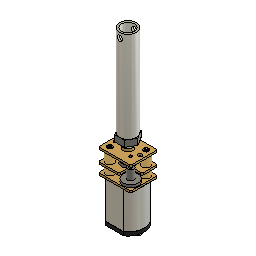
MicroGearMotor v14 (Autodesk Fusion 360 design; units mm, degrees)
Autodesk Fusion 360 part; units mm, degrees
note: some values were not read from the file. Chosen so that the rebuilt part matches the saved one: which bodies a step acts on; which face or edge a step refers to; how an offset face is resized; where a step starts. Set by a fixed rule: which sketch regions a step uses.
sketch "Sketch1" plane through (0, 0, 0) normal (0, 1, 0) x (1, 0, 0) in component "GearboxScaffolding"
  line L0 (6, -5) -> (-6, -5)
  line L1 (-6, -5) -> (-6, 5)
  line L2 (-6, 5) -> (6, 5)
  line L3 (6, 5) -> (6, -5)
  line L4 (6, -5) -> (-6, 5) construction
  line L5 (-6, -5) -> (6, 5) construction
  circle A0 centre (0, 5) radius 0.5
  line L6 (6, -5) -> (3, -5) construction
  line L7 (3, -5) -> (3, -2) construction
  line L8 (3, -2) -> (6, -2) construction
  line L9 (6, -2) -> (6, -5) construction
  circle A1 centre (3, -2) radius 0.5
  circle A2 centre (0, 0) radius 2.8346
  circle A3 centre (0, 0) radius 1.5
  line L10 (-6, 5) -> (-3, 5) construction
  line L11 (-3, 5) -> (-3, 2) construction
  line L12 (-3, 2) -> (-6, 2) construction
  line L13 (-6, 2) -> (-6, 5) construction
  circle A4 centre (-3, 2) radius 0.5
  line L14 (-6, 0) -> (-4.5, 0) construction
  line L15 (6, 0) -> (4.5, 0) construction
  circle A5 centre (4.5, 0) radius 0.75
  circle A6 centre (-4.5, 0) radius 0.75
  line L16 (-6, -5) -> (-3.9, -5) construction
  line L17 (-3.9, -5) -> (-3.9, -2.9) construction
  line L18 (-3.9, -2.9) -> (-6, -2.9) construction
  line L19 (-6, -2.9) -> (-6, -5) construction
  line L20 (6, 5) -> (3.9, 5) construction
  line L21 (3.9, 5) -> (3.9, 2.9) construction
  line L22 (3.9, 2.9) -> (6, 2.9) construction
  line L23 (6, 2.9) -> (6, 5) construction
  circle A7 centre (3.9, 2.9) radius 1
  circle A8 centre (-3.9, -2.9) radius 1
  circle A9 centre (3.9, 2.9) radius 1.5
  circle A10 centre (-3.9, -2.9) radius 1.5
  line L24 (-3.7, -3.6) -> (-4.1, -3.6)
  line L25 (-4.1, -3.6) -> (-4.1, -2.2)
  line L26 (-4.1, -2.2) -> (-3.7, -2.2)
  line L27 (-3.7, -2.2) -> (-3.7, -3.6)
  line L28 (-3.7, -3.6) -> (-4.1, -2.2) construction
  line L29 (-4.1, -3.6) -> (-3.7, -2.2) construction
  line L30 (-3.2, -3.1) -> (-4.6, -3.1)
  line L31 (-4.6, -3.1) -> (-4.6, -2.7)
  line L32 (-4.6, -2.7) -> (-3.2, -2.7)
  line L33 (-3.2, -2.7) -> (-3.2, -3.1)
  line L34 (-3.2, -3.1) -> (-4.6, -2.7) construction
  line L35 (-4.6, -3.1) -> (-3.2, -2.7) construction
  line L36 (4.6, 2.7) -> (3.2, 2.7)
  line L37 (3.2, 2.7) -> (3.2, 3.1)
  line L38 (3.2, 3.1) -> (4.6, 3.1)
  line L39 (4.6, 3.1) -> (4.6, 2.7)
  line L40 (4.6, 2.7) -> (3.2, 3.1) construction
  line L41 (3.2, 2.7) -> (4.6, 3.1) construction
  line L42 (4.1, 2.2) -> (3.7, 2.2)
  line L43 (3.7, 2.2) -> (3.7, 3.6)
  line L44 (3.7, 3.6) -> (4.1, 3.6)
  line L45 (4.1, 3.6) -> (4.1, 2.2)
  line L46 (4.1, 2.2) -> (3.7, 3.6) construction
  line L47 (3.7, 2.2) -> (4.1, 3.6) construction
  circle A11 centre (-3, 2) radius 2.4
  circle A12 centre (-3, 2) radius 0.771
  circle A13 centre (3, -2) radius 1.175
  circle A14 centre (3, -2) radius 2.8556
  circle A15 centre (0, 0) radius 0.75
  circle A16 centre (0, 0) radius 2.4306
  circle A17 centre (0, 0) radius 1.2056
  circle A18 centre (-3.9, -2.9) radius 0.65
  circle A19 centre (3.9, 2.9) radius 0.65
  line L48 (1.6386, -5) -> (1.6386, -1.6451)
  line L49 (2.6386, -0.6451) -> (6, -0.6451)
  arc A20 (2.6386, -0.6451) -> (1.6386, -1.6451) centre (2.6386, -1.6451) ccw
  circle A21 centre (0, 0) radius 0.5
  dimension "d1" = 12
  dimension "d2" = 10
  dimension "d3" = 1
  dimension "d4" = 3
  dimension "d5" = 3
  dimension "d6" = 1
  dimension "d8" = 3
  dimension "d9" = 3
  dimension "d10" = 3
  dimension "d11" = 1
  dimension "d12" = 1.5
  dimension "d13" = 1.5
  dimension "d14" = 1.5
  dimension "d15" = 1.5
  dimension "d16" = 2.1
  dimension "d17" = 2.1
  dimension "d18" = 2.1
  dimension "d19" = 2.1
  dimension "d20" = 2
  dimension "d21" = 2
  dimension "d22" = 3
  dimension "d23" = 3
  dimension "d24" = 1.4
  dimension "d25" = 0.4
  dimension "d26" = 1.4
  dimension "d27" = 0.4
  dimension "d28" = 1.4
  dimension "d29" = 0.4
  dimension "d30" = 1.4
  dimension "d31" = 0.4
  dimension "d36" = 1.5
  dimension "d37" = 4.8
  dimension "d38" = 2.35
  dimension "d39" = 1.3
  dimension "d40" = 1.3
  dimension "d46" = 1
  dimension "d50" = 1
  measures "d3" diameter of A0
  measures "d6" diameter of A1
  measures "d8" diameter of A3
  measures "d11" diameter of A4
  measures "d14" diameter of A5
  measures "d15" diameter of A6
  measures "d20" diameter of A7
  measures "d21" diameter of A8
  measures "d22" diameter of A9
  measures "d23" diameter of A10
  measures "d36" diameter of A15
  measures "d37" diameter of A11
  measures "d38" diameter of A13
  measures "d39" diameter of A18
  measures "d40" diameter of A19
  measures "d46" radius of A20
  measures "d50" diameter of A21
extrude "Extrude1" add sketch "Sketch1" along normal blind 0.75 contours L0 L3 A14 L48 L49 | L0 L1 L2 L3 A0 A2 A5 A6 A11 A14 L48 L49 | A2 A5 A13 A14 L48 L49 | A2 A14 L48 | A5 A14 L49 | A2 A14 A16 L48 | A2 A11 A14 A16 | A2 A13 A16 L48 | A5 A14 | A5 A14 L49 | A5 L49 | A12 | A2 A6 A11 | A2 A11 A16 | A3 A11 A14 A16 | A3 A14 A16 L48 A20 | A2 A13 | A2 A13 | A16 L48 A20 | A2 A5 A14 L49 | A6 A11 | A6 A11 | A3 A11 A16 | A2 A13 A16 L49 A20 | A2 A11 A14 A16 | A2 A14 A16 L49 A20 | A3 A11 A14 A16 | A4 | A7 | A8 | A9 | A10 | L24 L25 L27 A18 | L30 L32 L33 A18 | L30 L31 L32 A18 | L25 L26 L27 A18 | L36 L38 L39 A19 | L42 L43 L45 A19 | L43 L44 L45 A19 | L36 L37 L38 A19 makes body 1 in component "GearboxScaffolding"
extrude "Extrude3" add sketch "Sketch1" along normal blind 0.75 from surface at 3.6 separate body contours L0 L1 L2 L3 A0 A2 A5 A6 A11 A14 L48 L49 | A2 A14 L48 | A5 A14 L49 | A2 A14 A16 L48 | A2 A11 A14 A16 | L2 A0 | A5 A14 | A5 A14 L49 | A12 | A2 A6 A11 | A2 A11 A16 | A3 A11 A14 A16 | A3 A14 A16 L48 A20 | A2 A5 A14 L49 | A6 A11 | A6 A11 | A3 A11 A16 | A3 A14 A17 | A3 A11 A14 A17 | A2 A11 A14 A16 | A2 A14 A16 L49 A20 | A3 A11 | A3 A11 A14 A16 | A15 | A14 A17 | A14 A17 | A3 A11 A14 A17 | A7 | A8 | A9 | A10 | L24 L25 L27 A18 | L30 L32 L33 A18 | L30 L31 L32 A18 | L25 L26 L27 A18 | L36 L38 L39 A19 | L42 L43 L45 A19 | L43 L44 L45 A19 | L36 L37 L38 A19 picked at (-0.075, 4.7758) makes body 2 in component "GearboxScaffolding"
extrude "Extrude4" add sketch "Sketch1" along normal blind 0.75 from surface at 8.36 separate body contours L0 L3 A14 L48 L49 | L0 L1 L2 L3 A0 A2 A5 A6 A11 A14 L48 L49 | A2 A5 A13 A14 L48 L49 | A2 A14 L48 | A5 A14 L49 | A2 A14 A16 L48 | A2 A11 A14 A16 | A2 A13 A16 L48 | L2 A0 | A12 | A2 A6 A11 | A2 A11 A16 | A3 A11 A14 A16 | A3 A14 A16 L48 A20 | A2 A13 | A2 A13 | A16 L48 A20 | A2 A5 A14 L49 | A3 A11 A16 | A3 A14 A17 | A3 A11 A14 A17 | A2 A13 A16 L49 A20 | A2 A11 A14 A16 | A2 A14 A16 L49 A20 | A3 A11 | A3 A11 A14 A16 | A3 A11 A14 A17 | A7 | A8 | A9 | A10 | L24 L25 L27 A18 | L30 L32 L33 A18 | L30 L31 L32 A18 | L25 L26 L27 A18 | L36 L38 L39 A19 | L42 L43 L45 A19 | L43 L44 L45 A19 | L36 L37 L38 A19 picked at (5.3235, -0.5556) picked at (-0.075, 4.7758) makes body 3 in component "GearboxScaffolding"
extrude "Extrude5" add sketch "Sketch1" along normal blind 2.85 from surface at 0.75 separate body contours A9 | A10 makes body 4 at (-2.4019, 2.65, 2.9748) makes body 5 at (5.3981, 2.65, -2.8252) in component "GearboxScaffolding"
extrude "Extrude6" add sketch "Sketch1" along normal up to surface (4.01 mm away) from surface at 4.35 separate body contours A9 | A10 makes body 6 at (-2.4019, 7.0233, 2.9748) makes body 7 at (5.3981, 7.0233, -2.8252) in component "GearboxScaffolding"
extrude "Extrude7" add sketch "Sketch1" along normal blind 1 from surface at 0.85 separate body contours A2 A5 A13 A14 L48 L49 | A2 A14 L48 | A5 A14 L49 | A2 A14 A16 L48 | A2 A13 A16 L48 | A5 A14 L49 | A5 L49 | A3 A14 A16 L48 A20 | A2 A13 | A2 A13 | A16 L48 A20 | A2 A5 A14 L49 | A3 A14 A17 | A2 A13 A16 L49 A20 | A2 A14 A16 L49 A20 | A14 A17 picked at (0.8337, -0.3767) makes body 8 in component "GearboxScaffolding"
extrude "Extrude8" add sketch "Sketch1" along normal blind 3.65 from surface at 1.85 contours A2 A13 | A2 A13 bodies 8 in component "GearboxScaffolding"
extrude "Extrude9" add sketch "Sketch1" along normal up to surface (9.01 mm away) separate body contours A1 makes body 9 in component "GearboxScaffolding"
extrude "Extrude11" add sketch "Sketch1" along normal blind 1 from surface at 4.4 separate body contours A3 A11 A14 A16 | A3 A14 A16 L48 A20 | A16 L48 A20 | A3 A11 A16 | A3 A14 A17 | A3 A11 A14 A17 | A3 A11 | A3 A11 A14 A16 | A15 | A14 A17 | A14 A17 | A3 A11 A14 A17 makes body 10 in component "GearboxScaffolding"
extrude "Extrude12" add sketch "Sketch1" along normal blind 5 from surface at 3.7 separate body contours A21 makes body 11 in component "GearboxScaffolding"
extrude "Extrude13" add sketch "Sketch1" along normal blind 1 from surface at 5.4 contours A15 | A14 A17 | A14 A17 bodies 10 11 in component "GearboxScaffolding"
extrude "Extrude14" add sketch "Sketch1" along normal up to surface (5.31 mm away) from surface at 3.7 separate body contours A4 makes body 12 in component "GearboxScaffolding"
extrude "Extrude15" add sketch "Sketch1" along normal blind 1 from surface at 5.5 separate body contours A12 | A2 A6 A11 | A2 A11 A16 | A6 A11 | A3 A11 A16 | A3 A11 picked at (-4.3, 0.2493) makes body 13 in component "GearboxScaffolding"
extrude "Extrude16" add sketch "Sketch1" along normal blind 1.5 from surface at 6.5 separate body contours A12 makes body 14 in component "GearboxScaffolding"
extrude "Extrude17" add sketch "Sketch1" along normal blind 1.5 from surface at 6.6 contours A2 A14 A16 L48 | A2 A11 A14 A16 | A2 A13 A16 L48 | A2 A11 A16 | A3 A11 A14 A16 | A3 A14 A16 L48 A20 | A2 A13 | A16 L48 A20 | A3 A11 A16 | A3 A14 A17 | A3 A11 A14 A17 | A2 A13 A16 L49 A20 | A2 A11 A14 A16 | A2 A14 A16 L49 A20 | A3 A11 | A3 A11 A14 A16 | A15 | A14 A17 | A14 A17 | A3 A11 A14 A17 picked at (2.3463, -1.3388) bodies 10 14 in component "GearboxScaffolding"
extrude "Extrude18" add sketch "Sketch1" along normal blind 1 from surface at 9.11 contours A3 A14 A17 | A3 A11 A14 A17 | A3 A11 | A3 A11 A14 A17 bodies 3 in component "GearboxScaffolding"
extrude "Extrude19" add sketch "Sketch1" against normal blind 10.35 from surface at 9.11 separate body contours L25 L27 L30 A18 | L27 L30 A18 | L25 L30 A18 | L25 L27 L30 L32 | L27 L30 L32 A18 | L25 L30 L32 A18 | L25 L27 L32 A18 | L27 L32 A18 | L25 L32 A18 | L36 L45 A19 | L36 L38 L45 A19 | L36 L43 L45 A19 | L36 L38 L43 L45 | L38 L45 A19 | L36 L43 A19 | L36 L38 L43 A19 | L38 L43 L45 A19 | L38 L43 A19 makes body 15 at (-3.2532, 5.66, 2.8353) makes body 16 at (4.5468, 2.21, -2.8353) in component "GearboxScaffolding"
extrude "Extrude20" add sketch "Sketch1" against normal blind 1 draft -30 from surface at 9.11 contours A7 | A8 | L24 L25 L27 A18 | L25 L27 L30 A18 | L27 L30 A18 | L25 L30 A18 | L25 L27 L30 L32 | L27 L30 L32 A18 | L30 L32 L33 A18 | L25 L30 L32 A18 | L30 L31 L32 A18 | L25 L27 L32 A18 | L27 L32 A18 | L25 L32 A18 | L25 L26 L27 A18 | L36 L38 L39 A19 | L36 L45 A19 | L36 L38 L45 A19 | L36 L43 L45 A19 | L36 L38 L43 L45 | L42 L43 L45 A19 | L38 L45 A19 | L36 L43 A19 | L36 L38 L43 A19 | L38 L43 L45 A19 | L43 L44 L45 A19 | L36 L37 L38 A19 | L38 L43 A19 bodies 15 16 in component "GearboxScaffolding"
combine "Combine1" operation cut target body 3 tool bodies 15 16 keep tools in component "GearboxScaffolding"
extrude "Extrude21" cut sketch "Sketch1" against normal blind 0.2 draft -20 from surface at 9.11 contours L24 L25 L27 A18 | L25 L27 L30 A18 | L25 L27 L30 L32 | L27 L30 L32 A18 | L30 L32 L33 A18 | L25 L30 L32 A18 | L30 L31 L32 A18 | L25 L27 L32 A18 | L25 L26 L27 A18 | L36 L38 L39 A19 | L36 L38 L45 A19 | L36 L43 L45 A19 | L36 L38 L43 L45 | L42 L43 L45 A19 | L36 L38 L43 A19 | L38 L43 L45 A19 | L43 L44 L45 A19 | L36 L37 L38 A19 bodies 15 16 in component "GearboxScaffolding"
extrude "Extrude22" add sketch "Sketch1" along normal blind 35 from surface at 8.1 separate body contours A15 | A14 A17 | A14 A17 | A21 makes body 17 in component "GearboxScaffolding"
fillet "Fillet1" radius 0.5 13 edges at (6, 0.375, 5) (-6, 0.375, 5) (-6, 0.375, -5) (6, 0.375, -5) (6, 3.975, -5) (-6, 3.975, -5) (-6, 3.975, 5) (1.6386, 3.975, 5) (6, 3.975, 0.6451) (6, 8.735, 5) (-6, 8.735, 5) (-6, 8.735, -5) (6, 8.735, -5) on bodies 1 2 3 in component "GearboxScaffolding"
sketch "Sketch1 (2)" plane through (0, 0, 0) normal (0, 1, 0) x (1, 0, 0) in component "DC Motor"
  line L0 (6, -5) -> (-6, -5)
  line L1 (-6, -5) -> (-6, 5)
  line L2 (-6, 5) -> (6, 5)
  line L3 (6, 5) -> (6, -5)
  line L4 (6, -5) -> (-6, 5) construction
  line L5 (-6, -5) -> (6, 5) construction
  circle A0 centre (0, 0) radius 1.25
  circle A1 centre (0, 0) radius 6
  circle A2 centre (0, 0) radius 2
  circle A3 centre (0, -3.5) radius 0.5
  circle A4 centre (3.9, 2.9) radius 0.65
  circle A5 centre (-3.9, -2.9) radius 0.65
  circle A6 centre (0, 0) radius 0.75
  circle A7 centre (0, 0) radius 0.5
  circle A8 centre (0, 0) radius 2.5
  line L6 (-3.1659, -1.25) -> (-4.4659, -1.25)
  line L7 (-4.4659, -1.25) -> (-4.4659, 1.25)
  line L8 (-4.4659, 1.25) -> (-3.1659, 1.25)
  line L9 (-3.1659, 1.25) -> (-3.1659, -1.25)
  line L10 (-3.1659, -1.25) -> (-4.4659, 1.25) construction
  line L11 (-4.4659, -1.25) -> (-3.1659, 1.25) construction
  line L12 (0, 0) -> (0, 5) construction
  line L13 (3.1659, 1.25) -> (3.1659, -1.25)
  line L14 (4.4659, 1.25) -> (3.1659, 1.25)
  line L15 (4.4659, -1.25) -> (4.4659, 1.25)
  line L16 (3.1659, -1.25) -> (4.4659, -1.25)
  dimension "d108" = 12
  dimension "d109" = 10
  dimension "d112" = 2.5
  dimension "d113" = 4
  dimension "d114" = 1
  dimension "d115" = 3.5
  dimension "d130" = 5
  dimension "d131" = 2.5
  dimension "d132" = 1.3
  measures "d112" diameter of A0
  measures "d113" diameter of A2
  measures "d114" diameter of A3
  measures "d115" distance of A0.centre
  measures "d130" diameter of A8
extrude "Extrude1'" add sketch "Sketch1 (2)" against normal blind 13.75 separate body contours L0 L2 A1 | A0 | A2 | A3 | A4 | A5 | A6 | A7 | A8 | L6 L7 L8 L9 | L13 L14 L15 L16 makes body 18 in component "DC Motor"
extrude "Extrude2" add sketch "Sketch1 (2)" along normal blind 0.6 separate body contours A0 | A6 | A7 makes body 19 in component "DC Motor"
extrude "Extrude3'" add sketch "Sketch1 (2)" along normal blind 1.8 separate body contours A6 makes body 20 in component "DC Motor"
extrude "Extrude4'" add sketch "Sketch1 (2)" along normal blind 1.9 separate body contours A7 makes body 21 in component "DC Motor"
extrude "Extrude5'" cut sketch "Sketch1 (2)" against normal blind 2 contours A3 | A4 | A5 bodies 18 19 20 21 in component "DC Motor"
extrude "Extrude6'" add sketch "Sketch1 (2)" against normal blind 1.35 from surface at -13.75 separate body contours L0 L2 A1 | A2 | A3 | A4 | A5 | A8 | L6 L7 L8 L9 | L13 L14 L15 L16 makes body 22 in component "DC Motor"
move_face "OffsetFaces1" offset -0.05 6 faces at (1.1055, -14.2, 5) (4.3878, -14.65, 4.0923) (3.5474, -14.65, -4.839) (1.1055, -14.65, -5) (-3.5474, -14.2, -4.839) (-3.5474, -14.65, 4.839) on bodies 22 in component "DC Motor"
extrude "Extrude7'" add sketch "Sketch1 (2)" against normal blind 1.75 from surface at -15.1 separate body contours L6 L7 L8 L9 | L13 L14 L15 L16 makes body 23 at (-4.4659, -16.2667, 0.4167) makes body 24 at (4.4659, -16.2667, 0.4167) in component "DC Motor"
fillet "Fillet1'" radius 1.15 4 edges at (-3.8159, -16.85, 1.25) (-3.8159, -16.85, -1.25) (3.8159, -16.85, 1.25) (3.8159, -16.85, -1.25) on bodies 23 24 in component "DC Motor"
hole "Hole1" at (-4.4659, -15.8828, 0) direction (1, 0, 0) diameter 1 depth 8.932 tip angle 180 bodies 24 23 in component "DC Motor"
extrude "Extrude8'" add sketch "Sketch1 (2)" against normal blind 1 from surface at -15.1 contours A2 | A8 bodies 22 in component "DC Motor"
extrude "Extrude9'" add sketch "Sketch1 (2)" against normal blind 2 from surface at -13.75 separate body contours A0 | A6 | A7 makes body 25 in component "DC Motor"
thread "Thread1" "ISO Metric profile 3.0 M3x0.5 6g" major diameter 2.927 minor diameter 2.3555 pitch 0.5 angle 60 resizes the face on face at (1.2, 31.4333, -0.1153) on bodies 17 in component "GearboxScaffolding"
move_face "OffsetFaces1'" offset 0.2 1 faces at (1.4981, 9.4433, -0.0748) on bodies 3 in component "GearboxScaffolding"
sketch "Sketch1 (3)" plane through (0, 0, 0) normal (0, 1, 0) x (1, 0, 0) in component "LeadNut"
  line L0 (1.8158, -3.145) -> (3.6315, 0)
  line L1 (3.6315, 0) -> (1.8158, 3.145)
  line L2 (1.8158, 3.145) -> (-1.8158, 3.145)
  line L3 (-1.8158, 3.145) -> (-3.6315, 0)
  line L4 (-3.6315, 0) -> (-1.8158, -3.145)
  line L5 (-1.8158, -3.145) -> (1.8158, -3.145)
  circle A0 centre (0, 0) radius 1.4546
extrude "Extrude1''" add sketch "Sketch1 (3)" along normal blind 2.32 separate body makes body 26 in component "LeadNut"
sketch "Sketch2" plane through (0, 2.32, 0) normal (0, 1, 0) x (-1, 0, 0) in component "LeadNut"
  circle A0 centre (0, 0) radius 1.4546
  line L0 (1.8158, 3.145) -> (-1.8158, 3.145)
  line L1 (-1.8158, 3.145) -> (-3.6315, 0)
  line L2 (-3.6315, 0) -> (-1.8158, -3.145)
  line L3 (-1.8158, -3.145) -> (1.8158, -3.145)
  line L4 (1.8158, -3.145) -> (3.6315, 0)
  line L5 (3.6315, 0) -> (1.8158, 3.145)
  circle A1 centre (0, 0) radius 3.145
  circle A2 centre (0, 0) radius 2.395
  dimension "d151" = 0.75
  measures "d151" distance of A1 A2
extrude "Extrude2'" add sketch "Sketch2" along normal blind 34 separate body contours A1 makes body 27 in component "LeadNut"
sketch "Sketch3" plane through (0, 0, 0) normal (0, 0, 1) x (1, 0, 0) in component "LeadNut"
  circle A0 centre (0, 34.4051) radius 1
  dimension "d154" = 2
  measures "d154" diameter of A0
extrude "Extrude3''" cut sketch "Sketch3" along normal through all and the other way through all bodies 27 in component "LeadNut"
sketch "Sketch1 (4)" plane through (0, 0, 0) normal (0, 1, 0) x (1, 0, 0)
component "GearboxScaffolding" placed x (1, 0, 0) y (0, 1, 0) z (0, 0, 1) at (0, -0.01, 0)
component "DC Motor" placed x (1, 0, 0) y (0, 1, 0) z (0, 0, 1) at (0, 0, 0)
component "LeadNut" placed x (1, 0, 0) y (0, 1, 0) z (0, 0, 1) at (0, 10.6601, 0)
